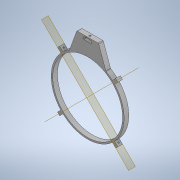
# Autodesk Inventor part: mount
Saved by Autodesk Inventor 2021.1 (Build 251245010, 245A)
## iProperties
Created: 2020-07-16
Part Number: mount
Material: PET Plastic
Document SubType Name: Modeling
Designer: robst
Density: 1.541 g/cm^3
Appearance: Light Gray
Author: robst
Autodesk Inventor part; units mm, degrees
ref_plane "YZ Plane" through (0, 0, 0) normal (1, 0, 0) x (0, 1, 0)
ref_plane "XY Plane" through (0, 0, 0) normal (0, 0, 1) x (1, 0, 0)
sketch "Sketch1" plane through (0, 0, 0) normal (0, 0, 1) x (1, 0, 0)
  circle A0 centre (0, 0) radius 142.875
  circle A1 centre (0, 0) radius 149.225
  dimension "innerDiameter" = 285.75
  dimension "outerDiameter" = 298.45
  constraints: 2 centre point, 2 coincident
  measures "innerDiameter" diameter of A0
  measures "outerDiameter" diameter of A1
extrude "Extrusion1" add sketch "Sketch1" along normal mid plane 19.05
sketch "Sketch2" plane through (0, 0, 0) normal (0, 0, 1) x (1, 0, 0)
  circle A0 centre (0, 0) radius 142.875 construction
  line L0 (0, 142.875) -> (0, 149.225) construction
  circle A1 centre (0, 0) radius 149.225 construction
  line L1 (0, 142.875) -> (44.45, 142.875)
  line L2 (44.45, 142.875) -> (44.45, 149.225)
  line L3 (44.45, 149.225) -> (19.05, 149.225)
  line L4 (0, 142.875) -> (-44.45, 142.875)
  line L5 (-44.45, 142.875) -> (-44.45, 149.225)
  line L6 (-44.45, 149.225) -> (19.05, 149.225)
  line L7 (371.6693, 35.081) -> (0, 0)
  dimension "halfBaseWidth" = 44.45
  dimension "baseThickness" = 6.35
  dimension "baseHeight" = 0
  constraints: 16 end point, 2 perpendicular, 2 symmetric about line, 2 vertical alignment, 1 horizontal, 1 point on line, 1 vertical, 2 other
  measures "halfBaseWidth" distance of L1.start L1.end
  measures "baseThickness" distance of L1.end L2.end
  measures "baseHeight" distance of L1.start L0.start
extrude "Extrusion2" add sketch "Sketch2" along normal mid plane 19.05
sketch "Sketch5" plane through (-44.45, 149.225, 9.525) normal (0, 1, 0) x (1, 0, 0)
  line L0 (0, 19.05) -> (0, 0) projected
  line L1 (88.9, 19.05) -> (88.9, 0) projected
  line L2 (0, 0) -> (88.9, 0)
  line L3 (88.9, 0) -> (88.9, 19.05)
  line L4 (88.9, 19.05) -> (0, 19.05)
  line L5 (0, 19.05) -> (0, 0)
  point P0 (44.45, 9.525)
  point P1 (0, 19.05)
  constraints: 8 end point, 2 parallel, 1 horizontal, 1 perpendicular
extrude "Extrusion3" add sketch "Sketch5" along normal blind 63.5
sketch "Sketch7" plane through (0, 0, 9.525) normal (0, 0, 1) x (1, 0, 0)
  line L0 (-44.45, 142.875) -> (-44.45, 212.725) projected
  line L1 (-44.45, 212.725) -> (44.45, 212.725) projected
  line L2 (44.45, 142.875) -> (44.45, 212.725) projected
  line L3 (0, 212.725) -> (0, 149.1868) construction
  line L4 (-15.875, 197.104) -> (15.875, 197.104)
  line L5 (15.875, 197.104) -> (15.875, 206.375)
  line L6 (15.875, 206.375) -> (-15.875, 206.375)
  line L7 (-15.875, 206.375) -> (-15.875, 197.104)
  line L8 (-15.875, 197.104) -> (15.875, 206.375) construction
  line L9 (15.875, 197.104) -> (-15.875, 206.375) construction
  point P0 (0, 0)
  point P1 (-38.1, 144.2792)
  point P2 (38.1, 144.2792)
  point P3 (0, 201.7395)
  dimension "screwHoleWidth" = 31.75
  dimension "screwHoleHeight" = 9.271
  dimension "screwHoleSupportThickness" = 6.35
  constraints: 14 end point, 3 midpoint, 2 parallel, 2 perpendicular, 1 point on line, 2 other
  measures "screwHoleWidth" distance of L4.start L4.end
  measures "screwHoleHeight" distance of L5.end L4.end
  measures "screwHoleSupportThickness" distance between parallel lines of L6 L1
extrude "Extrusion4" cut sketch "Sketch7" against normal through all
sketch "Sketch6" plane through (-44.45, 212.725, 9.525) normal (0, 1, 0) x (1, 0, 0)
  point P0 (44.45, 9.525)
  point P1 (44.45, 9.525)
  constraints: 1 coincident
hole "Hole2" at (0, 212.725, 0) direction (0, -1, 0) diameter 6.7564 depth 6.35 tip angle 118 clearance for "Flat Head Machine Screw (82)" size "1/4" standard "Ansi Unified Screw Threads"
ref_plane "Work Plane1" through (0, 0, 0) normal (-0.7071068, 0.7071068, 0) x (0, 0, 1)
ref_plane "Work Plane2" through (0, 0, 0) normal (0.7071068, 0.7071068, 0) x (0, 0, 1)
sketch "Sketch11" plane through (0, 0, 0) normal (0, 0, 1) x (1, 0, 0)
  arc A0 (-43.0678, 142.875) -> (43.0678, 142.875) centre (0, 0) ccw projected
  circle A1 centre (0, 0) radius 142.875 projected
  line L0 (-214.9625, 214.9625) -> (217.3313, -217.3313) projected
  line L1 (-101.0279, 101.0279) -> (-96.5378, 105.518)
  line L2 (-101.0279, 101.0279) -> (-94.6779, 101.0279) construction
  line L3 (-96.5378, 105.518) -> (-114.4983, 123.4785)
  line L4 (-96.5378, 105.518) -> (-71.1378, 105.518) construction
  line L5 (-114.4983, 123.4785) -> (-118.9884, 118.9884)
  line L6 (-118.9884, 118.9884) -> (-101.0279, 101.0279)
  line L7 (-101.0279, 101.0279) -> (-105.518, 96.5378)
  line L8 (-105.518, 96.5378) -> (-123.4785, 114.4983)
  line L9 (-123.4785, 114.4983) -> (-118.9884, 118.9884)
  point P0 (38.1, 144.2792)
  point P1 (-38.1, 144.2792)
  point P2 (-109.9126, 100.9323)
  point P3 (-100.9323, 109.9126)
  dimension "d47" = 6.35
  dimension "d48" = 45
  dimension "d49" = 25.4
  dimension "d50" = 135
  constraints: 18 end point, 3 perpendicular, 2 equal length, 2 horizontal, 2 point on line, 2 symmetric about line, 3 other
  measures "d47" distance of L1.start L1.end
  measures "d48" angle of L2 L1
  measures "d49" distance of L1.end L3.end
  measures "d50" angle of L4 L3
extrude "Extrusion7" add sketch "Sketch11" along normal mid plane 19.05 contours A0 L0 L5 L3 | A0 L8 L9 L0
sketch "Sketch12" plane through (-114.4983, 123.4785, -9.525) normal (0.7071068, 0.7071068, 0) x (-0.7071068, 0.7071068, 0)
  line L0 (0, 0) -> (0, 19.05) projected
  line L1 (-19.1852, 19.05) -> (0, 19.05) projected
  line L2 (-19.1852, 0) -> (-19.1852, 19.05) projected
  line L3 (0, 0) -> (-19.1852, 0) projected
  line L4 (-9.5926, 19.05) -> (-9.5926, 0) construction
  line L5 (0, 9.525) -> (-19.1852, 9.525) construction
  point P0 (-168.275, 9.525)
  point P1 (-9.5926, 9.525)
  constraints: 5 midpoint, 4 end point
hole "Hole4" at (-107.7153, 116.6955, 0) direction (-0.7071068, -0.7071068, 0) diameter 5.1054 depth 12.7 tip angle 118 clearance for "Flat Head Machine Screw (82)" size "#10" standard "Ansi Unified Screw Threads"
pattern_circular "Circular Pattern1" count 4 over 360 about axis through (0, 0, -10) along (0, 0, 1) of "Extrusion7", "Hole4"
sketch "Sketch13" plane through (0, 0, 9.525) normal (0, 0, 1) x (1, 0, 0)
  line L0 (-15.875, 206.375) -> (15.875, 206.375) projected
  line L1 (-44.45, 212.725) -> (44.45, 212.725) projected
  line L2 (0, 208.915) -> (8.89, 208.915)
  line L3 (8.89, 208.915) -> (8.89, 206.375)
  line L4 (8.89, 206.375) -> (0, 206.375)
  line L5 (0, 208.915) -> (0, 206.375)
  line L6 (15.875, 206.375) -> (-15.875, 206.375)
  line L7 (0, 208.915) -> (-8.89, 208.915)
  line L8 (-8.89, 208.915) -> (-8.89, 206.375)
  point P0 (0, 0)
  dimension "d63" = 8.89
  dimension "d64" = 2.54
  constraints: 14 end point, 4 symmetric about line, 2 point on line, 1 horizontal, 1 midpoint, 1 perpendicular, 1 vertical
  measures "d63" distance of L2.start L2.end
  measures "d64" distance of L2.end L3.end
extrude "Extrusion8" cut sketch "Sketch13" against normal through all
sketch "Sketch14" plane through (0, 0, 9.525) normal (0, 0, 1) x (1, 0, 0)
  point P0 (0, 0)
sketch "Sketch15" plane through (0, 0, 0) normal (0, 0, 1) x (1, 0, 0)
  arc A0 (-43.0678, 142.875) -> (-100.9323, 109.9126) centre (0, 0) ccw projected
  line L0 (-43.0678, 142.875) -> (-44.45, 142.875) projected
  line L1 (44.45, 142.875) -> (43.0678, 142.875) projected
  arc A1 (100.9323, 109.9126) -> (43.0678, 142.875) centre (0, 0) ccw projected
  line L2 (-44.45, 142.875) -> (-44.45, 142.451)
  line L3 (-44.45, 142.875) -> (-43.0678, 142.875)
  line L4 (43.0678, 142.875) -> (44.45, 142.875)
  line L5 (44.45, 142.875) -> (44.45, 142.451)
  arc A2 (-43.0678, 142.875) -> (-44.45, 142.451) centre (0, 0) ccw
  arc A3 (44.45, 142.451) -> (43.0678, 142.875) centre (0, 0) ccw
  constraints: 8 end point, 5 point on circle, 2 centre point, 1 coincident, 1 horizontal, 1 perpendicular, 1 vertical
extrude "Extrusion9" add sketch "Sketch15" along normal mid plane 19.05
sketch "Sketch16" plane through (0, 0, 0) normal (0, 0, 1) x (1, 0, 0)
  line L0 (44.45, 142.451) -> (44.45, 212.725) projected
  line L1 (-44.45, 142.451) -> (-44.45, 212.725) projected
  arc A0 (-44.45, 142.451) -> (-100.9323, 109.9126) centre (0, 0) ccw projected
  arc A1 (100.9323, 109.9126) -> (44.45, 142.451) centre (0, 0) ccw projected
  line L2 (0, 0) -> (-74.6125, 129.2326) construction
  line L3 (0, 0) -> (0, 149.225) construction
  line L4 (0, 0) -> (74.6125, 129.2326) construction
  line L5 (-44.45, 212.725) -> (-74.6125, 129.2326)
  line L6 (-44.45, 142.451) -> (-44.45, 212.725) projected
  line L7 (-44.45, 142.451) -> (-44.45, 212.725)
  line L8 (44.45, 212.725) -> (44.45, 142.451)
  line L9 (44.45, 212.725) -> (74.6125, 129.2326)
  arc A2 (74.6125, 129.2326) -> (44.45, 142.451) centre (0, 0) ccw
  arc A3 (-44.45, 142.451) -> (-74.6125, 129.2326) centre (0, 0) ccw
  dimension "d69" = 30
  dimension "d70" = 30
  constraints: 14 end point, 4 point on circle, 2 centre point, 2 vertical, 1 coincident, 1 collinear, 1 point on line
  measures "d69" angle of L2 L3
  measures "d70" angle of L4 L3
extrude "Extrusion10" add sketch "Sketch16" along normal mid plane 19.05
fillet "Fillet1" radius 3.175 2 edges at (-74.6125, 129.2326, 0) (74.6125, 129.2326, 0)
fillet "Fillet2" radius 3.175 2 edges at (-44.45, 212.725, 0) (44.45, 212.725, 0)
equation "\"outerDiameter\" = innerDiameter + 2 * ringThicknessRadius"
equation "\"d7\" = ringWidth"
equation "\"d51\" = ringWidth"
equation "\"d67\" = ringWidth"
equation "\"d71\" = ringWidth"
equation "\"ringThicknessRadius\" = 6.35"
equation "\"ringWidth\" = 19.05"
body "Solid1"
